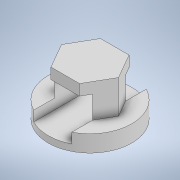
# Autodesk Inventor part: Деталь
Saved by Autodesk Inventor 2021 (Build 250183000, 183)
## iProperties
Created: 2021-11-21
Part Number: Деталь
Material: Типовые
Document SubType Name: Modeling
Designer: jmiha
Density: 1 g/cm^3
Appearance: По умолчанию
Author: jmiha
Autodesk Inventor part; units mm, degrees
ref_plane "YZ Plane" through (0, 0, 0) normal (1, 0, 0) x (0, 1, 0)
ref_plane "XZ Plane" through (0, 0, 0) normal (0, 1, 0) x (-1, 0, 0)
ref_plane "XY Plane" through (0, 0, 0) normal (0, 0, 1) x (1, 0, 0)
sketch "Эскиз1" plane through (0, 0, 0) normal (0, 1, 0) x (-1, 0, 0)
  circle A0 centre (0, 0) radius 50
  dimension "d0" = 100
  constraints: 1 centre point, 1 coincident
  measures "d0" diameter of A0
extrude "Выдавливание1" add sketch "Эскиз1" along normal blind 20
sketch "Эскиз2" plane through (0, 20, 0) normal (0, 1, 0) x (1, 0, 0)
  line L0 (17.0801, 29.5836) -> (34.1603, 0)
  line L1 (34.1603, 0) -> (17.0801, -29.5836)
  line L2 (17.0801, -29.5836) -> (-17.0801, -29.5836)
  line L3 (-17.0801, -29.5836) -> (-34.1603, 0)
  line L4 (-34.1603, 0) -> (-17.0801, 29.5836)
  line L5 (-17.0801, 29.5836) -> (17.0801, 29.5836)
  point P0 (0, 0)
  point P1 (0, 0)
  constraints: 12 end point, 1 coincident, 1 horizontal, 13 other
extrude "Выдавливание2" add sketch "Эскиз2" along normal blind 40
sketch "Эскиз3" plane through (0, 0, 0) normal (0, 0, 1) x (1, 0, 0)
  line L0 (-22.8201, 7.7625) -> (22.8201, 7.7625)
  line L1 (22.8201, 7.7625) -> (22.8201, 46.9937)
  line L2 (22.8201, 46.9937) -> (-22.8201, 46.9937)
  line L3 (-22.8201, 46.9937) -> (-22.8201, 7.7625)
  line L4 (-22.8201, 7.7625) -> (22.8201, 46.9937) construction
  line L5 (22.8201, 7.7625) -> (-22.8201, 46.9937) construction
  point P0 (0, 0)
  point P1 (0, 27.3781)
  constraints: 12 end point, 2 midpoint, 2 parallel, 1 horizontal, 1 perpendicular
extrude "Выдавливание3" cut sketch "Эскиз3" against normal through all both and the other way through all
sketch "Эскиз4" plane through (0, 0, 0) normal (1, 0, 0) x (0, 1, 0)
  point P0 (0, 0)
